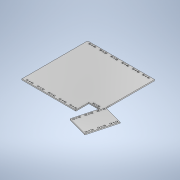
# Autodesk Inventor part: base_plate
Saved by Autodesk Inventor 2020.1 (Build 241239000, 239)
## iProperties
Created: 2019-07-16
Part Number: base_plate
Material: Générique
Document SubType Name: Modeling
Designer: Thibault
Density: 1 g/cm^3
Appearance: Aluminum - Poli
Author: Thibault
Autodesk Inventor part; units mm, degrees
ref_plane "YZ Plane" through (0, 0, 0) normal (1, 0, 0) x (0, 1, 0)
ref_plane "XZ Plane" through (0, 0, 0) normal (0, 1, 0) x (-1, 0, 0)
ref_plane "XY Plane" through (0, 0, 0) normal (0, 0, 1) x (1, 0, 0)
sketch "Anchor (screw side)" plane through (0, 0, 0) normal (0, 0, 1) x (1, 0, 0)
  circle A0 centre (93.8994, 50.3042) radius 1.05
  line L0 (90.8494, 51.3542) -> (87.7494, 51.3542)
  line L1 (87.7494, 51.3542) -> (87.7494, 49.2542)
  line L2 (87.7494, 49.2542) -> (90.8494, 49.2542)
  line L3 (90.8494, 49.2542) -> (90.8494, 51.3542)
  line L4 (100.0494, 51.3542) -> (96.9494, 51.3542)
  line L5 (96.9494, 51.3542) -> (96.9494, 49.2542)
  line L6 (96.9494, 49.2542) -> (100.0494, 49.2542)
  line L7 (100.0494, 49.2542) -> (100.0494, 51.3542)
  line L8 (90.8494, 51.3542) -> (96.9494, 49.2542) construction
  line L9 (96.9494, 51.3542) -> (90.8494, 49.2542) construction
  line L10 (85.7494, 53.3542) -> (102.0494, 53.3542) construction
  line L11 (102.0494, 53.3542) -> (102.0494, 47.2542) construction
  line L12 (102.0494, 47.2542) -> (85.7494, 47.2542) construction
  line L13 (85.7494, 47.2542) -> (85.7494, 53.3542) construction
  point P0 (103.5798, 50.1132)
  dimension "d27" = 2.1
  dimension "d28" = 3.1
  dimension "d29" = 2.1
  dimension "slot_distance" = 6.1
  dimension "d34" = 2
  dimension "d35" = 2
  dimension "d36" = 2
  dimension "d37" = 2
  measures "d27" diameter of A0
  measures "d28" distance of L2.end L1.end
  measures "d29" distance of L1.end L0.end
  measures "slot_distance" distance between parallel lines of L5 L3
  measures "d34" distance between parallel lines of L0 L10
  measures "d35" distance between parallel lines of L12 L2
  measures "d36" distance between parallel lines of L11 L7
  measures "d37" distance between parallel lines of L13 L1
sketch "Anchor (nut side)" plane through (0, 0, 0) normal (0, 0, 1) x (1, 0, 0)
  line L0 (11.1, 0) -> (9.1, 0)
  line L1 (9.1, 0) -> (9.1, -2)
  line L2 (9.1, -2) -> (9.9, -2)
  line L3 (9.9, -2) -> (9.9, -4)
  line L4 (6.2, -4) -> (6.2, -2)
  line L5 (6.2, -2) -> (7, -2)
  line L6 (7, -2) -> (7, 0)
  line L7 (7, 0) -> (5, 0)
  line L8 (2, 0) -> (2, 2)
  line L9 (2, 0) -> (3, 0) construction
  line L10 (2, 2) -> (5, 2)
  line L11 (5, 2) -> (5, 0)
  line L12 (11.1, 0) -> (11.1, 2)
  line L13 (11.1, 2) -> (14.1, 2)
  line L14 (14.1, 2) -> (14.1, 0)
  line L15 (0, 0) -> (2, 0)
  line L16 (14.1, 0) -> (16.1, 0)
  line L17 (6.2, -4) -> (7, -4)
  line L18 (9.9, -4) -> (9.1, -4)
  line L19 (7, -4) -> (7, -6.25)
  line L20 (9.1, -4) -> (9.1, -6.25)
  line L21 (7.25, -6.5) -> (8.05, -6.5)
  arc A0 (7, -6.25) -> (7.25, -6.5) centre (7.25, -6.25) ccw
  arc A1 (8.85, -6.5) -> (9.1, -6.25) centre (8.85, -6.25) ccw
  line L22 (8.05, -6.5) -> (8.85, -6.5)
  line L23 (8.05, -3.8983) -> (8.05, -9.959) construction
  point P0 (9.1321, -0.6227)
  point P1 (7, -6.5)
  point P2 (9.1, -6.5)
  dimension "d3" = 2
  dimension "d7" = 6.1
  dimension "d10" = 2
  dimension "d11" = 2
  dimension "d12" = 0.8
  dimension "d13" = 2
  dimension "d14" = 0.8
  dimension "d15" = 2.1
  dimension "d18" = 2
  dimension "d19" = 0.8
  dimension "d20" = 0.8
  dimension "d21" = 2.5
  dimension "d22" = 2.5
  dimension "d23" = 2.1
  dimension "d38" = 2
  dimension "d39" = 0.25
  dimension "d120" = 3
  measures "d3" distance of L15.start L8.start
  measures "d7" distance of L7.end L0.start
  measures "d10" distance of L0.start L0.end
  measures "d11" distance of L0.end L1.end
  measures "d12" distance of L1.end L2.end
  measures "d13" distance of L2.end L3.end
  measures "d14" distance of L4.end L5.end
  measures "d15" distance of L6.end L0.end
  measures "d18" distance of L14.end L16.end
  measures "d19" distance of L4.start L17.end
  measures "d20" distance of L3.end L18.end
  measures "d21" distance of L17.end point (7, -6.5)
  measures "d22" distance of L18.end point (9.1, -6.5)
  measures "d23" distance of L17.end L18.end
  measures "d38" distance between parallel lines of L15 L10
  measures "d39" radius of A0
  measures "d120" distance of L8.end L10.end
derived "shared_parameters.ipt"
sketch "Esquisse2" plane through (0, 0, 0) normal (0, 1, 0) x (-1, 0, 0)
  line L0 (-79.4831, 87.8462) -> (-182.2224, 87.8462)
  line L1 (-206.9471, 55.6654) -> (-206.9471, -37.2538)
  line L2 (-206.9471, -37.2538) -> (-81.4831, -37.2538)
  line L3 (-79.4831, -35.2538) -> (-79.4831, 87.8462)
  line L4 (-81.4831, -37.2538) -> (-79.4831, -35.2538)
  line L5 (-243.956, 65.5819) -> (-229.8504, 118.2248)
  line L6 (-229.8504, 118.2248) -> (-191.1168, 107.8462)
  line L7 (-191.1168, 107.8462) -> (-205.2224, 55.2032)
  line L8 (-205.2224, 55.2032) -> (-243.956, 65.5819)
  line L9 (-182.2224, 63.1426) -> (-203.0951, 63.1426)
  line L10 (-182.2224, 87.8462) -> (-182.2224, 63.1426)
  line L11 (-116.4758, 87.8462) -> (-191.1168, 107.8462)
  circle A0 centre (-91.2922, -34.2038) radius 1.05
  line L12 (-94.3422, -33.1538) -> (-97.4422, -33.1538)
  line L13 (-97.4422, -33.1538) -> (-97.4422, -35.2538)
  line L14 (-97.4422, -35.2538) -> (-94.3422, -35.2538)
  line L15 (-94.3422, -35.2538) -> (-94.3422, -33.1538)
  line L16 (-85.1422, -33.1538) -> (-88.2422, -33.1538)
  line L17 (-88.2422, -33.1538) -> (-88.2422, -35.2538)
  line L18 (-88.2422, -35.2538) -> (-85.1422, -35.2538)
  line L19 (-85.1422, -35.2538) -> (-85.1422, -33.1538)
  line L20 (-94.3422, -33.1538) -> (-88.2422, -35.2538) construction
  line L21 (-88.2422, -33.1538) -> (-94.3422, -35.2538) construction
  line L22 (-99.4422, -31.1538) -> (-83.1422, -31.1538) construction
  line L23 (-83.1422, -31.1538) -> (-83.1422, -37.2538) construction
  line L24 (-83.1422, -37.2538) -> (-99.4422, -37.2538) construction
  line L25 (-99.4422, -37.2538) -> (-99.4422, -31.1538) construction
  circle A1 centre (-112.2821, -34.2038) radius 1.05
  line L26 (-115.3321, -33.1538) -> (-118.4321, -33.1538)
  line L27 (-118.4321, -33.1538) -> (-118.4321, -35.2538)
  line L28 (-118.4321, -35.2538) -> (-115.3321, -35.2538)
  line L29 (-115.3321, -35.2538) -> (-115.3321, -33.1538)
  line L30 (-106.1321, -33.1538) -> (-109.2321, -33.1538)
  line L31 (-109.2321, -33.1538) -> (-109.2321, -35.2538)
  line L32 (-109.2321, -35.2538) -> (-106.1321, -35.2538)
  line L33 (-106.1321, -35.2538) -> (-106.1321, -33.1538)
  line L34 (-115.3321, -33.1538) -> (-109.2321, -35.2538) construction
  line L35 (-109.2321, -33.1538) -> (-115.3321, -35.2538) construction
  line L36 (-120.4321, -31.1538) -> (-104.1321, -31.1538) construction
  line L37 (-104.1321, -31.1538) -> (-104.1321, -37.2538) construction
  line L38 (-104.1321, -37.2538) -> (-120.4321, -37.2538) construction
  line L39 (-120.4321, -37.2538) -> (-120.4321, -31.1538) construction
  circle A2 centre (-133.2392, -34.2038) radius 1.05
  line L40 (-136.2892, -33.1538) -> (-139.3892, -33.1538)
  line L41 (-139.3892, -33.1538) -> (-139.3892, -35.2538)
  line L42 (-139.3892, -35.2538) -> (-136.2892, -35.2538)
  line L43 (-136.2892, -35.2538) -> (-136.2892, -33.1538)
  line L44 (-127.0892, -33.1538) -> (-130.1892, -33.1538)
  line L45 (-130.1892, -33.1538) -> (-130.1892, -35.2538)
  line L46 (-130.1892, -35.2538) -> (-127.0892, -35.2538)
  line L47 (-127.0892, -35.2538) -> (-127.0892, -33.1538)
  line L48 (-136.2892, -33.1538) -> (-130.1892, -35.2538) construction
  line L49 (-130.1892, -33.1538) -> (-136.2892, -35.2538) construction
  line L50 (-141.3892, -31.1538) -> (-125.0892, -31.1538) construction
  line L51 (-125.0892, -31.1538) -> (-125.0892, -37.2538) construction
  line L52 (-125.0892, -37.2538) -> (-141.3892, -37.2538) construction
  line L53 (-141.3892, -37.2538) -> (-141.3892, -31.1538) construction
  circle A3 centre (-153.9202, -34.2038) radius 1.05
  line L54 (-156.9702, -33.1538) -> (-160.0702, -33.1538)
  line L55 (-160.0702, -33.1538) -> (-160.0702, -35.2538)
  line L56 (-160.0702, -35.2538) -> (-156.9702, -35.2538)
  line L57 (-156.9702, -35.2538) -> (-156.9702, -33.1538)
  line L58 (-147.7702, -33.1538) -> (-150.8702, -33.1538)
  line L59 (-150.8702, -33.1538) -> (-150.8702, -35.2538)
  line L60 (-150.8702, -35.2538) -> (-147.7702, -35.2538)
  line L61 (-147.7702, -35.2538) -> (-147.7702, -33.1538)
  line L62 (-156.9702, -33.1538) -> (-150.8702, -35.2538) construction
  line L63 (-150.8702, -33.1538) -> (-156.9702, -35.2538) construction
  line L64 (-162.0702, -31.1538) -> (-145.7702, -31.1538) construction
  line L65 (-145.7702, -31.1538) -> (-145.7702, -37.2538) construction
  line L66 (-145.7702, -37.2538) -> (-162.0702, -37.2538) construction
  line L67 (-162.0702, -37.2538) -> (-162.0702, -31.1538) construction
  circle A4 centre (-174.0724, -34.2038) radius 1.05
  line L68 (-177.1224, -33.1538) -> (-180.2224, -33.1538)
  line L69 (-180.2224, -33.1538) -> (-180.2224, -35.2538)
  line L70 (-180.2224, -35.2538) -> (-177.1224, -35.2538)
  line L71 (-177.1224, -35.2538) -> (-177.1224, -33.1538)
  line L72 (-167.9224, -33.1538) -> (-171.0224, -33.1538)
  line L73 (-171.0224, -33.1538) -> (-171.0224, -35.2538)
  line L74 (-171.0224, -35.2538) -> (-167.9224, -35.2538)
  line L75 (-167.9224, -35.2538) -> (-167.9224, -33.1538)
  line L76 (-177.1224, -33.1538) -> (-171.0224, -35.2538) construction
  line L77 (-171.0224, -33.1538) -> (-177.1224, -35.2538) construction
  line L78 (-182.2224, -31.1538) -> (-165.9224, -31.1538) construction
  line L79 (-165.9224, -31.1538) -> (-165.9224, -37.2538) construction
  line L80 (-165.9224, -37.2538) -> (-182.2224, -37.2538) construction
  line L81 (-182.2224, -37.2538) -> (-182.2224, -31.1538) construction
  circle A5 centre (-193.4497, -34.2038) radius 1.05
  line L82 (-196.4997, -33.1538) -> (-199.5997, -33.1538)
  line L83 (-199.5997, -33.1538) -> (-199.5997, -35.2538)
  line L84 (-199.5997, -35.2538) -> (-196.4997, -35.2538)
  line L85 (-196.4997, -35.2538) -> (-196.4997, -33.1538)
  line L86 (-187.2997, -33.1538) -> (-190.3997, -33.1538)
  line L87 (-190.3997, -33.1538) -> (-190.3997, -35.2538)
  line L88 (-190.3997, -35.2538) -> (-187.2997, -35.2538)
  line L89 (-187.2997, -35.2538) -> (-187.2997, -33.1538)
  line L90 (-196.4997, -33.1538) -> (-190.3997, -35.2538) construction
  line L91 (-190.3997, -33.1538) -> (-196.4997, -35.2538) construction
  line L92 (-201.5997, -31.1538) -> (-185.2997, -31.1538) construction
  line L93 (-185.2997, -31.1538) -> (-185.2997, -37.2538) construction
  line L94 (-185.2997, -37.2538) -> (-201.5997, -37.2538) construction
  line L95 (-201.5997, -37.2538) -> (-201.5997, -31.1538) construction
  circle A6 centre (-91.2922, 84.7962) radius 1.05
  line L96 (-94.3422, 85.8462) -> (-97.4422, 85.8462)
  line L97 (-97.4422, 85.8462) -> (-97.4422, 83.7462)
  line L98 (-97.4422, 83.7462) -> (-94.3422, 83.7462)
  line L99 (-94.3422, 83.7462) -> (-94.3422, 85.8462)
  line L100 (-85.1422, 85.8462) -> (-88.2422, 85.8462)
  line L101 (-88.2422, 85.8462) -> (-88.2422, 83.7462)
  line L102 (-88.2422, 83.7462) -> (-85.1422, 83.7462)
  line L103 (-85.1422, 83.7462) -> (-85.1422, 85.8462)
  line L104 (-94.3422, 85.8462) -> (-88.2422, 83.7462) construction
  line L105 (-88.2422, 85.8462) -> (-94.3422, 83.7462) construction
  line L106 (-99.4422, 87.8462) -> (-83.1422, 87.8462) construction
  line L107 (-83.1422, 87.8462) -> (-83.1422, 81.7462) construction
  line L108 (-83.1422, 81.7462) -> (-99.4422, 81.7462) construction
  line L109 (-99.4422, 81.7462) -> (-99.4422, 87.8462) construction
  circle A7 centre (-112.2821, 84.7962) radius 1.05
  line L110 (-115.3321, 85.8462) -> (-118.4321, 85.8462)
  line L111 (-118.4321, 85.8462) -> (-118.4321, 83.7462)
  line L112 (-118.4321, 83.7462) -> (-115.3321, 83.7462)
  line L113 (-115.3321, 83.7462) -> (-115.3321, 85.8462)
  line L114 (-106.1321, 85.8462) -> (-109.2321, 85.8462)
  line L115 (-109.2321, 85.8462) -> (-109.2321, 83.7462)
  line L116 (-109.2321, 83.7462) -> (-106.1321, 83.7462)
  line L117 (-106.1321, 83.7462) -> (-106.1321, 85.8462)
  line L118 (-115.3321, 85.8462) -> (-109.2321, 83.7462) construction
  line L119 (-109.2321, 85.8462) -> (-115.3321, 83.7462) construction
  line L120 (-120.4321, 87.8462) -> (-104.1321, 87.8462) construction
  line L121 (-104.1321, 87.8462) -> (-104.1321, 81.7462) construction
  line L122 (-104.1321, 81.7462) -> (-120.4321, 81.7462) construction
  line L123 (-120.4321, 81.7462) -> (-120.4321, 87.8462) construction
  circle A8 centre (-133.2392, 84.7962) radius 1.05
  line L124 (-136.2892, 85.8462) -> (-139.3892, 85.8462)
  line L125 (-139.3892, 85.8462) -> (-139.3892, 83.7462)
  line L126 (-139.3892, 83.7462) -> (-136.2892, 83.7462)
  line L127 (-136.2892, 83.7462) -> (-136.2892, 85.8462)
  line L128 (-127.0892, 85.8462) -> (-130.1892, 85.8462)
  line L129 (-130.1892, 85.8462) -> (-130.1892, 83.7462)
  line L130 (-130.1892, 83.7462) -> (-127.0892, 83.7462)
  line L131 (-127.0892, 83.7462) -> (-127.0892, 85.8462)
  line L132 (-136.2892, 85.8462) -> (-130.1892, 83.7462) construction
  line L133 (-130.1892, 85.8462) -> (-136.2892, 83.7462) construction
  line L134 (-141.3892, 87.8462) -> (-125.0892, 87.8462) construction
  line L135 (-125.0892, 87.8462) -> (-125.0892, 81.7462) construction
  line L136 (-125.0892, 81.7462) -> (-141.3892, 81.7462) construction
  line L137 (-141.3892, 81.7462) -> (-141.3892, 87.8462) construction
  circle A9 centre (-153.9202, 84.7962) radius 1.05
  line L138 (-156.9702, 85.8462) -> (-160.0702, 85.8462)
  line L139 (-160.0702, 85.8462) -> (-160.0702, 83.7462)
  line L140 (-160.0702, 83.7462) -> (-156.9702, 83.7462)
  line L141 (-156.9702, 83.7462) -> (-156.9702, 85.8462)
  line L142 (-147.7702, 85.8462) -> (-150.8702, 85.8462)
  line L143 (-150.8702, 85.8462) -> (-150.8702, 83.7462)
  line L144 (-150.8702, 83.7462) -> (-147.7702, 83.7462)
  line L145 (-147.7702, 83.7462) -> (-147.7702, 85.8462)
  line L146 (-156.9702, 85.8462) -> (-150.8702, 83.7462) construction
  line L147 (-150.8702, 85.8462) -> (-156.9702, 83.7462) construction
  line L148 (-162.0702, 87.8462) -> (-145.7702, 87.8462) construction
  line L149 (-145.7702, 87.8462) -> (-145.7702, 81.7462) construction
  line L150 (-145.7702, 81.7462) -> (-162.0702, 81.7462) construction
  line L151 (-162.0702, 81.7462) -> (-162.0702, 87.8462) construction
  circle A10 centre (-174.0724, 84.7962) radius 1.05
  line L152 (-177.1224, 85.8462) -> (-180.2224, 85.8462)
  line L153 (-180.2224, 85.8462) -> (-180.2224, 83.7462)
  line L154 (-180.2224, 83.7462) -> (-177.1224, 83.7462)
  line L155 (-177.1224, 83.7462) -> (-177.1224, 85.8462)
  line L156 (-167.9224, 85.8462) -> (-171.0224, 85.8462)
  line L157 (-171.0224, 85.8462) -> (-171.0224, 83.7462)
  line L158 (-171.0224, 83.7462) -> (-167.9224, 83.7462)
  line L159 (-167.9224, 83.7462) -> (-167.9224, 85.8462)
  line L160 (-177.1224, 85.8462) -> (-171.0224, 83.7462) construction
  line L161 (-171.0224, 85.8462) -> (-177.1224, 83.7462) construction
  line L162 (-182.2224, 87.8462) -> (-165.9224, 87.8462) construction
  line L163 (-165.9224, 87.8462) -> (-165.9224, 81.7462) construction
  line L164 (-165.9224, 81.7462) -> (-182.2224, 81.7462) construction
  line L165 (-182.2224, 81.7462) -> (-182.2224, 87.8462) construction
  circle A11 centre (-193.4497, 60.0926) radius 1.05
  line L166 (-196.4997, 61.1426) -> (-199.5997, 61.1426)
  line L167 (-199.5997, 61.1426) -> (-199.5997, 59.0426)
  line L168 (-199.5997, 59.0426) -> (-196.4997, 59.0426)
  line L169 (-196.4997, 59.0426) -> (-196.4997, 61.1426)
  line L170 (-187.2997, 61.1426) -> (-190.3997, 61.1426)
  line L171 (-190.3997, 61.1426) -> (-190.3997, 59.0426)
  line L172 (-190.3997, 59.0426) -> (-187.2997, 59.0426)
  line L173 (-187.2997, 59.0426) -> (-187.2997, 61.1426)
  line L174 (-196.4997, 61.1426) -> (-190.3997, 59.0426) construction
  line L175 (-190.3997, 61.1426) -> (-196.4997, 59.0426) construction
  line L176 (-201.5997, 63.1426) -> (-185.2997, 63.1426) construction
  line L177 (-185.2997, 63.1426) -> (-185.2997, 57.0426) construction
  line L178 (-185.2997, 57.0426) -> (-201.5997, 57.0426) construction
  line L179 (-201.5997, 57.0426) -> (-201.5997, 63.1426) construction
  circle A12 centre (-238.9006, 72.6648) radius 1.05
  line L180 (-237.097, 75.3391) -> (-236.2946, 78.3335)
  line L181 (-236.2946, 78.3335) -> (-238.3231, 78.877)
  line L182 (-238.3231, 78.877) -> (-239.1254, 75.8826)
  line L183 (-239.1254, 75.8826) -> (-237.097, 75.3391)
  line L184 (-239.4781, 66.4526) -> (-238.6758, 69.4469)
  line L185 (-238.6758, 69.4469) -> (-240.7042, 69.9905)
  line L186 (-240.7042, 69.9905) -> (-241.5065, 66.9961)
  line L187 (-241.5065, 66.9961) -> (-239.4781, 66.4526)
  line L188 (-237.097, 75.3391) -> (-240.7042, 69.9905) construction
  line L189 (-238.6758, 69.4469) -> (-239.1254, 75.8826) construction
  line L190 (-233.8451, 79.7477) -> (-238.0639, 64.0031) construction
  line L191 (-238.0639, 64.0031) -> (-243.956, 65.5819) construction
  line L192 (-243.956, 65.5819) -> (-239.7373, 81.3265) construction
  line L193 (-239.7373, 81.3265) -> (-233.8451, 79.7477) construction
  circle A13 centre (-233.9571, 91.114) radius 1.05
  line L194 (-232.1535, 93.7883) -> (-231.3512, 96.7826)
  line L195 (-231.3512, 96.7826) -> (-233.3796, 97.3262)
  line L196 (-233.3796, 97.3262) -> (-234.182, 94.3318)
  line L197 (-234.182, 94.3318) -> (-232.1535, 93.7883)
  line L198 (-234.5347, 84.9017) -> (-233.7323, 87.8961)
  line L199 (-233.7323, 87.8961) -> (-235.7608, 88.4396)
  line L200 (-235.7608, 88.4396) -> (-236.5631, 85.4453)
  line L201 (-236.5631, 85.4453) -> (-234.5347, 84.9017)
  line L202 (-232.1535, 93.7883) -> (-235.7608, 88.4396) construction
  line L203 (-233.7323, 87.8961) -> (-234.182, 94.3318) construction
  line L204 (-228.9017, 98.1969) -> (-233.1204, 82.4523) construction
  line L205 (-233.1204, 82.4523) -> (-239.0126, 84.0311) construction
  line L206 (-239.0126, 84.0311) -> (-234.7938, 99.7756) construction
  line L207 (-234.7938, 99.7756) -> (-228.9017, 98.1969) construction
  circle A14 centre (-229.0137, 109.5631) radius 1.05
  line L208 (-227.2101, 112.2375) -> (-226.4077, 115.2318)
  line L209 (-226.4077, 115.2318) -> (-228.4362, 115.7753)
  line L210 (-228.4362, 115.7753) -> (-229.2385, 112.781)
  line L211 (-229.2385, 112.781) -> (-227.2101, 112.2375)
  line L212 (-229.5912, 103.3509) -> (-228.7889, 106.3453)
  line L213 (-228.7889, 106.3453) -> (-230.8173, 106.8888)
  line L214 (-230.8173, 106.8888) -> (-231.6197, 103.8945)
  line L215 (-231.6197, 103.8945) -> (-229.5912, 103.3509)
  line L216 (-227.2101, 112.2375) -> (-230.8173, 106.8888) construction
  line L217 (-228.7889, 106.3453) -> (-229.2385, 112.781) construction
  line L218 (-223.9582, 116.646) -> (-228.177, 100.9014) construction
  line L219 (-228.177, 100.9014) -> (-234.0691, 102.4802) construction
  line L220 (-234.0691, 102.4802) -> (-229.8504, 118.2248) construction
  line L221 (-229.8504, 118.2248) -> (-223.9582, 116.646) construction
  circle A15 centre (-206.0591, 63.8649) radius 1.05
  line L222 (-204.2555, 66.5392) -> (-203.4531, 69.5336)
  line L223 (-203.4531, 69.5336) -> (-205.4816, 70.0771)
  line L224 (-205.4816, 70.0771) -> (-206.2839, 67.0828)
  line L225 (-206.2839, 67.0828) -> (-204.2555, 66.5392)
  line L226 (-206.6366, 57.6527) -> (-205.8343, 60.6471)
  line L227 (-205.8343, 60.6471) -> (-207.8627, 61.1906)
  line L228 (-207.8627, 61.1906) -> (-208.6651, 58.1962)
  line L229 (-208.6651, 58.1962) -> (-206.6366, 57.6527)
  line L230 (-204.2555, 66.5392) -> (-207.8627, 61.1906) construction
  line L231 (-205.8343, 60.6471) -> (-206.2839, 67.0828) construction
  line L232 (-201.0037, 70.9478) -> (-205.2224, 55.2032) construction
  line L233 (-205.2224, 55.2032) -> (-211.1146, 56.782) construction
  line L234 (-211.1146, 56.782) -> (-206.8958, 72.5266) construction
  line L235 (-206.8958, 72.5266) -> (-201.0037, 70.9478) construction
  circle A16 centre (-201.1157, 82.3141) radius 1.05
  line L236 (-199.312, 84.9884) -> (-198.5097, 87.9828)
  line L237 (-198.5097, 87.9828) -> (-200.5381, 88.5263)
  line L238 (-200.5381, 88.5263) -> (-201.3405, 85.5319)
  line L239 (-201.3405, 85.5319) -> (-199.312, 84.9884)
  line L240 (-201.6932, 76.1019) -> (-200.8908, 79.0963)
  line L241 (-200.8908, 79.0963) -> (-202.9193, 79.6398)
  line L242 (-202.9193, 79.6398) -> (-203.7216, 76.6454)
  line L243 (-203.7216, 76.6454) -> (-201.6932, 76.1019)
  line L244 (-199.312, 84.9884) -> (-202.9193, 79.6398) construction
  line L245 (-200.8908, 79.0963) -> (-201.3405, 85.5319) construction
  line L246 (-196.0602, 89.397) -> (-200.279, 73.6524) construction
  line L247 (-200.279, 73.6524) -> (-206.1711, 75.2312) construction
  line L248 (-206.1711, 75.2312) -> (-201.9524, 90.9758) construction
  line L249 (-201.9524, 90.9758) -> (-196.0602, 89.397) construction
  circle A17 centre (-196.1722, 100.7633) radius 1.05
  line L250 (-194.3686, 103.4376) -> (-193.5663, 106.432)
  line L251 (-193.5663, 106.432) -> (-195.5947, 106.9755)
  line L252 (-195.5947, 106.9755) -> (-196.397, 103.9811)
  line L253 (-196.397, 103.9811) -> (-194.3686, 103.4376)
  line L254 (-196.7497, 94.5511) -> (-195.9474, 97.5455)
  line L255 (-195.9474, 97.5455) -> (-197.9758, 98.089)
  line L256 (-197.9758, 98.089) -> (-198.7782, 95.0946)
  line L257 (-198.7782, 95.0946) -> (-196.7497, 94.5511)
  line L258 (-194.3686, 103.4376) -> (-197.9758, 98.089) construction
  line L259 (-195.9474, 97.5455) -> (-196.397, 103.9811) construction
  line L260 (-191.1168, 107.8462) -> (-195.3355, 92.1016) construction
  line L261 (-195.3355, 92.1016) -> (-201.2277, 93.6804) construction
  line L262 (-201.2277, 93.6804) -> (-197.0089, 109.425) construction
  line L263 (-197.0089, 109.425) -> (-191.1168, 107.8462) construction
  point P0 (0, 0)
  point P1 (-79.4831, -37.2538)
  dimension "d5" = 20.99
  dimension "d6" = 20.9571
  dimension "d8" = 20.681
  dimension "d9" = 20.1522
  dimension "d16" = 19.3773
  dimension "d41" = 96.3965
  dimension "d42" = 19.1
  dimension "d43" = 19.1
  dimension "d44" = 34
  dimension "d49" = 121.1
  dimension "d17" = 13.4974
  dimension "d24" = 11.8091
  dimension "d33" = 2
  dimension "d40" = 2
  dimension "angle" = 105
  dimension "dist_b" = 20
  dimension "dist_a" = 23
  constraints: 24 end point, 13 horizontal, 5 point on line, 4 parallel, 2 perpendicular, 2 vertical, 1 collinear, 4 other
  measures "d33" distance of L2.end point (-79.483, -37.254)
  measures "d40" distance of L3.start point (-79.483, -37.254)
  measures "angle" angle of L8 L10
  measures "dist_b" vertical distance of L6.end L0.end
  measures "dist_a" distance from line of L10 L7.end
extrude "Extrusion2" add sketch "Esquisse2" along normal blind 2 contours L3 L4 L2 L1 L8 L7 L9 L10 L0 | L7 L8 L5 L6
equation "\"d5\" = kws_bp_anchor_dist6"
equation "\"d6\" = kws_bp_anchor_dist5"
equation "\"d8\" = kws_bp_anchor_dist4"
equation "\"d9\" = kws_bp_anchor_dist3"
equation "\"d16\" = kws_bp_anchor_dist2"
equation "\"d41\" = short_switchplate_depth + extra_slot_dim"
equation "\"d42\" = tc_anchor_dist"
equation "\"d43\" = tc_anchor_dist"
equation "\"d44\" = tc_plates_dist"
equation "\"d17\" = kws_bp_anchor_dist1"
equation "\"d24\" = kws_bp_anchor_dist7"
equation "\"d40\" = d33"
equation "\"d25\" = sheet_thickness"
equation "\"kws_bp_anchor_dist6\" = 20.989963"
equation "\"kws_bp_anchor_dist5\" = 20.957075"
equation "\"kws_bp_anchor_dist4\" = 20.680968"
equation "\"kws_bp_anchor_dist3\" = 20.15222"
equation "\"kws_bp_anchor_dist2\" = 19.377291"
equation "\"short_switchplate_depth\" = 96.296447"
equation "\"extra_slot_dim\" = 0.1"
equation "\"tc_anchor_dist\" = 19.1"
equation "\"tc_plates_dist\" = 34"
equation "\"kws_bp_anchor_dist1\" = 13.497405"
equation "\"kws_bp_anchor_dist7\" = 11.809109"
equation "\"sheet_thickness\" = 2"
